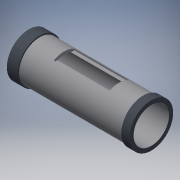
# Autodesk Inventor part: Handle bars holder axle
Saved by Autodesk Inventor 2018 (Build 220112000, 112)
## iProperties
Created: 2018-08-14
Part Number: Handle bars holder axle
Material: Generic
Document SubType Name: Modeling
Designer: ruben
Density: 1 g/cm^3
Appearance: Default
Author: ruben
Autodesk Inventor part; units mm, degrees
ref_plane "YZ Plane" through (0, 0, 0) normal (1, 0, 0) x (0, 1, 0)
ref_plane "XY Plane" through (0, 0, 0) normal (0, 0, 1) x (1, 0, 0)
sketch "Sketch1" plane through (0, 0, 0) normal (0, 1, 0) x (-1, 0, 0)
  line L0 (-12.6, 0) -> (-15.4, 0) projected
  line L1 (0, -53.2) -> (0, 53.2) projected
  line L2 (-13, -38) -> (-15, -38)
  line L3 (-15, -38) -> (-15, 38)
  line L4 (-15, 38) -> (-13, 38)
  line L5 (-13, 38) -> (-13, -38)
  line L6 (-13, -38) -> (-15, 38) construction
  line L7 (-15, -38) -> (-13, 38) construction
  point P0 (-14, 0)
  dimension "d0" = 2
  dimension "d1" = 76
  dimension "d2" = 30
  constraints: 12 end point, 3 midpoint, 2 parallel, 1 horizontal, 1 perpendicular
  measures "d0" distance of L3.end L4.end
  measures "d1" distance of L2.end L3.end
  measures "d2" diameter of L3 L1
revolve "Revolution1" add sketch "Sketch1" angle 360 about axis through (0, 0, -10) along (0, 0, 1)
ref_plane "Work Plane1" through (0, 15, 0) normal (0, 1, 0) x (-1, 0, 0)
sketch "Sketch3" plane through (0, 15, 0) normal (0, 1, 0) x (-1, 0, 0)
  line L0 (-7.5, -20) -> (7.5, -20)
  line L1 (7.5, -20) -> (7.5, 20)
  line L2 (7.5, 20) -> (-7.5, 20)
  line L3 (-7.5, 20) -> (-7.5, -20)
  line L4 (-7.5, -20) -> (7.5, 20) construction
  line L5 (7.5, -20) -> (-7.5, 20) construction
  point P0 (0, 0)
  dimension "d4" = 15
  dimension "d5" = 40
  constraints: 12 end point, 2 midpoint, 2 parallel, 1 horizontal, 1 perpendicular
  measures "d4" distance of L2.end L1.end
  measures "d5" distance of L1.end L0.end
extrude "Extrusion1" cut sketch "Sketch3" against normal blind 3
sketch "Sketch5" plane through (0, 0, -38) normal (0, 0, -1) x (-1, 0, 0)
  circle A0 centre (0, 0) radius 13
  circle A1 centre (0, 0) radius 16
  dimension "d8" = 32
  dimension "d9" = 26
  constraints: 2 centre point, 2 coincident
  measures "d8" diameter of A1
  measures "d9" diameter of A0
extrude "Extrusion2" add sketch "Sketch5" along normal blind 8
sketch "Sketch6" plane through (0, 0, 38) normal (0, 0, 1) x (1, 0, 0)
  circle A0 centre (0, 0) radius 13
  circle A1 centre (0, 0) radius 16
  dimension "d12" = 26
  dimension "d13" = 32
  constraints: 2 centre point, 2 coincident
  measures "d12" diameter of A0
  measures "d13" diameter of A1
extrude "Extrusion3" add sketch "Sketch6" along normal blind 6
body "Solid1"
